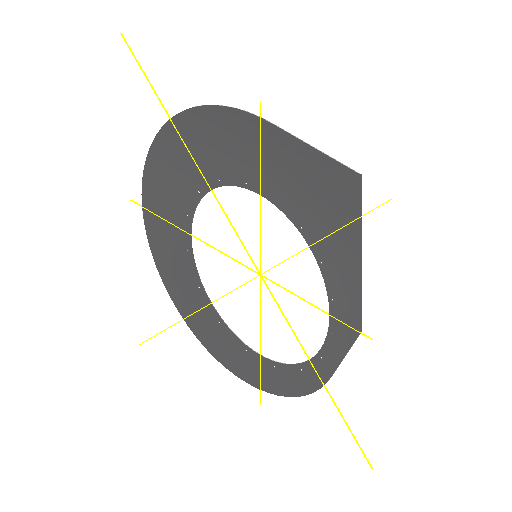
# Autodesk Inventor part: inlet side sheet
Saved by Autodesk Inventor 2022 (Build 260148000, 148)
## iProperties
Created: 2007-05-11
Part Number: inlet side sheet
Material: Steel, Mild
Document SubType Name: Modeling
Designer: LionelF
Density: 7.86 g/cm^3
Mass: 22171.9 g
Surface Area: 17999.4 cm^2
Volume: 2820.85 cm^3
Appearance: Steel
Author: LionelF
Autodesk Inventor part; units mm, degrees
ref_plane "YZ Plane" through (0, 0, 0) normal (1, 0, 0) x (0, 1, 0)
ref_plane "XZ Plane" through (0, 0, 0) normal (0, 1, 0) x (-1, 0, 0)
ref_plane "XY Plane" through (0, 0, 0) normal (0, 0, 1) x (1, 0, 0)
sketch "Sketch1" plane through (0, 0, 0) normal (0, 0, 1) x (1, 0, 0)
  circle A0 centre (0, 0) radius 69.85 construction
  line L0 (69.85, 0) -> (34.925, -60.4919) construction
  line L1 (34.925, -60.4919) -> (-34.925, -60.4919) construction
  line L2 (-34.925, -60.4919) -> (-69.85, 0) construction
  line L3 (-69.85, 0) -> (-34.925, 60.4919) construction
  line L4 (-34.925, 60.4919) -> (34.925, 60.4919) construction
  line L5 (34.925, 60.4919) -> (69.85, 0) construction
  line L6 (69.85, 0) -> (69.85, 777.875) construction
  line L7 (0, 60.4919) -> (0, -60.4919) construction
  line L8 (-69.85, 0) -> (69.85, 0) construction
  arc A1 (69.85, 777.875) -> (-319.0875, 673.6595) centre (69.85, 0) ccw
  arc A2 (-319.0875, 673.6595) -> (-673.1, 60.4919) centre (34.925, 60.4919) ccw
  arc A3 (-673.1, 60.4919) -> (-354.0125, -492.1839) centre (-34.925, 60.4919) ccw
  arc A4 (-354.0125, -492.1839) -> (214.3125, -492.1839) centre (-69.85, 0) ccw
  arc A5 (214.3125, -492.1839) -> (463.55, -60.4919) centre (-34.925, -60.4919) ccw
  arc A6 (463.55, -60.4919) -> (458.7952, 3.175) centre (34.925, -60.4919) ccw
  line L9 (458.7952, 3.175) -> (571.5, 3.175)
  line L10 (571.5, 3.175) -> (571.5, 777.875)
  line L11 (69.85, 777.875) -> (571.5, 777.875)
  line L12 (571.5, 3.175) -> (400.325, -303.4625)
  dimension "d0" = 777.875
  dimension "d1" = 139.7
  dimension "d2" = 571.5
  dimension "d3" = 774.7
  dimension "d5" = 498.475
  constraints: 27 end point, 17 point on circle, 7 centre point, 7 coincident, 3 midpoint, 3 perpendicular, 2 tangent, 1 horizontal, 1 vertical, 11 other
  measures "d0" distance of L0.start L6.end
  measures "d1" diameter of A0
  measures "d2" distance between parallel lines of L10 L7
  measures "d3" distance of L9.end L10.end
  measures "d5" radius of A5
extrude "Extrusion1" add sketch "Sketch1" along normal blind 3.175
hole "Hole1" at (0, 0, 0) direction (0, 0, 1) diameter 784.225 end through all
ref_plane "Work Plane1" through (0, 0, 1833.3831) normal (-1, 0, 0) x (0, 0, 1)
ref_plane "Work Plane2" through (0, 0, 1833.3831) normal (0, -1, 0) x (0, 0, 1)
ref_plane "Work Plane3" through (0, 0, 1833.3831) normal (0.7071, -0.7071, 0) x (0, 0, 1)
ref_plane "Work Plane4" through (0, 0, 1833.3831) normal (-0.7071, -0.7071, 0) x (0, 0, 1)
sketch "Sketch2" plane through (0, 0, 3.175) normal (0, 0, 1) x (1, 0, 0)
  circle A0 centre (0, 0) radius 392.1125 projected
  point P0 (411.0471, 81.7624)
  dimension "d19" = 419.1
  dimension "d20" = 81.7623
  measures "d19" distance of A0.centre point (411.047, 81.762)
  measures "d20" vertical distance of A0.centre point (411.047, 81.762)
hole "Hole2" at (411.0471, 81.7624, 3.175) direction (0, 0, -1) diameter 9.525 end through all
pattern_circular "Circular Pattern1" count 16 over 360 about axis through (0, 0, 1833.3831) along (0, 0, 1) of "Hole2"
equation "\"d20\" = 0.19509 * d19"
body "Solid1"
